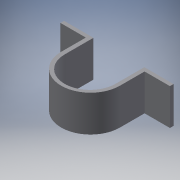
# Autodesk Inventor part: enganche eje muñeca
Saved by Autodesk Inventor 2016 (Build 200138000, 138)
## iProperties
Created: 2016-07-27
Part Number: enganche eje muñeca
Material: Generic
Document SubType Name: Modeling
Designer: Admin
Density: 1 g/cm^3
Appearance: Default
Author: Admin
Autodesk Inventor part; units mm, degrees
ref_plane "YZ Plane" through (0, 0, 0) normal (1, 0, 0) x (0, 1, 0)
ref_plane "XZ Plane" through (0, 0, 0) normal (0, 1, 0) x (-1, 0, 0)
ref_plane "XY Plane" through (0, 0, 0) normal (0, 0, 1) x (1, 0, 0)
sketch "Sketch1" plane through (0, 0, 0) normal (0, 0, 1) x (1, 0, 0)
  arc A0 (-183.89, 145.1838) -> (-169.84, 145.1838) centre (-176.865, 145.0255) ccw
  line L0 (-169.84, 145.1838) -> (-183.89, 145.1838) construction
  arc A1 (-184.9979, 145.368) -> (-168.7803, 145.1838) centre (-176.8902, 145.1838) ccw
  line L1 (-183.89, 145.1838) -> (-185, 145.1838)
  line L2 (-169.84, 145.1838) -> (-168.7803, 145.1838)
  line L3 (-168.7803, 145.1838) -> (-169.84, 145.1838)
  line L4 (-169.84, 145.1838) -> (-169.84, 152.9838)
  line L5 (-169.84, 152.9838) -> (-168.7803, 152.9838)
  line L6 (-168.7803, 152.9838) -> (-168.7803, 145.1838)
  line L7 (-185, 145.1838) -> (-183.89, 145.1838)
  line L8 (-183.89, 145.1838) -> (-183.89, 152.9838)
  line L9 (-183.89, 152.9838) -> (-185, 152.9838)
  line L10 (-185, 152.9838) -> (-185, 145.1838)
  line L11 (-168.7803, 152.9838) -> (-161.7803, 152.9838)
  line L12 (-161.7803, 152.9838) -> (-161.7803, 151.9838)
  line L13 (-161.7803, 151.9838) -> (-168.7803, 151.9838)
  line L14 (-168.7803, 151.9838) -> (-168.7803, 152.9838)
  line L15 (-185, 152.9838) -> (-192, 152.9838)
  line L16 (-192, 152.9838) -> (-192, 151.9838)
  line L17 (-192, 151.9838) -> (-185, 151.9838)
  line L18 (-185, 151.9838) -> (-185, 152.9838)
  point P0 (0, 0)
  dimension "d0" = 14.05
  dimension "d12" = 7.8
  dimension "d13" = 7.8
  dimension "d14" = 1
  dimension "d15" = 7
  dimension "d16" = 1
  dimension "d17" = 7
  constraints: 38 end point, 8 parallel, 5 point on circle, 4 horizontal, 4 perpendicular, 2 centre point, 1 collinear
  measures "d0" distance of L0.start L0.end
  measures "d12" distance of L3.end L4.end
  measures "d13" distance of L8.end L7.end
  measures "d14" distance of L11.end L12.end
  measures "d15" distance of L17.end L16.end
  measures "d16" distance of L16.end L15.end
  measures "d17" distance of L12.end L13.end
extrude "Extrusion2" add sketch "Sketch1" along normal blind 10
body "Solid2"
